Autodesk Fusion 360 part; units mm, degrees
note: some values were not read from the file. Chosen so that the rebuilt part matches the saved one: a side; which face or edge a step refers to. Set by a fixed rule: which sketch regions a step uses.
(part 2 of 2)
sketch "Sketch19" plane through (0, -4, 0) normal (0, -1, 0) x (1, 0, 0)
  line L0 (6.8, -6.4133) -> (7.8, -7.4133)
  line L1 (7.8, -7.4133) -> (11.75, -7.4133)
  line L2 (11.75, -7.4133) -> (11.75, -18.4133)
  line L3 (11.75, -18.4133) -> (0.75, -18.4133)
  line L4 (0.75, -18.4133) -> (0.75, -7.4133)
  line L5 (0.75, -7.4133) -> (4.7, -7.4133)
  line L6 (4.7, -7.4133) -> (5.7, -6.4133)
  line L7 (5.7, -6.4133) -> (5.7, 19.65)
  line L8 (5.7, 19.65) -> (6.8, 19.65)
  line L9 (6.8, 19.65) -> (6.8, -6.4133)
  arc A0 (25.83, 39.15) -> (20.83, 44.15) centre (20.83, 39.15) ccw
  line L10 (20.83, 44.15) -> (-20.83, 44.15)
  arc A1 (-20.83, 44.15) -> (-25.83, 39.15) centre (-20.83, 39.15) ccw
  line L11 (-25.83, 39.15) -> (-25.83, -22)
  arc A2 (-25.83, -22) -> (-20.83, -27) centre (-20.83, -22) ccw
  line L12 (-20.83, -27) -> (20.83, -27)
  arc A3 (20.83, -27) -> (25.83, -22) centre (20.83, -22) ccw
  line L13 (25.83, -22) -> (25.83, 39.15)
  line L14 (-15, 37.7778) -> (-15, 39)
  line L15 (-15, 39) -> (15, 39)
  line L16 (15, 39) -> (15, 37.7778)
  line L17 (15, 37.7778) -> (-15, 37.7778)
  circle A4 centre (20.83, 39.15) radius 1.5
  circle A5 centre (20.83, -22) radius 1.5
  circle A6 centre (-20.83, 39.15) radius 1.5
  circle A7 centre (-20.83, -22) radius 1.5
  line L18 (-5.7, -6.4133) -> (-4.7, -7.4133)
  line L19 (-4.7, -7.4133) -> (-0.75, -7.4133)
  line L20 (-0.75, -7.4133) -> (-0.75, -18.4133)
  line L21 (-0.75, -18.4133) -> (-11.75, -18.4133)
  line L22 (-11.75, -18.4133) -> (-11.75, -7.4133)
  line L23 (-11.75, -7.4133) -> (-7.8, -7.4133)
  line L24 (-7.8, -7.4133) -> (-6.8, -6.4133)
  line L25 (-6.8, -6.4133) -> (-6.8, 19.65)
  line L26 (-6.8, 19.65) -> (-5.7, 19.65)
  line L27 (-5.7, 19.65) -> (-5.7, -6.4133)
  line L28 (-6.8, -6.4133) -> (-5.7, -6.4133)
  line L29 (-8.8, -6.4133) -> (-8.8, 21.65) construction
  line L30 (-8.8, 21.65) -> (-3.7, 21.65) construction
  line L31 (-3.7, 21.65) -> (-3.7, -6.4133) construction
  line L32 (-8.8, -6.4133) -> (-8.8, -7.4133)
  line L33 (-3.7, -6.4133) -> (-3.7, -7.4133)
  line L34 (-7.8, -7.4133) -> (-4.7, -7.4133) construction
  line L35 (0, -27) -> (0, 44.15) construction
  line L36 (-3.7, -7.4133) -> (-8.8, -7.4133)
  line L37 (-8.8, -7.4133) -> (-8.8, 21.65)
  line L38 (-8.8, 21.65) -> (-3.7, 21.65)
  line L39 (-3.7, 21.65) -> (-3.7, -7.4133)
  line L40 (8.8, -7.4133) -> (8.8, 21.65)
  line L41 (8.8, 21.65) -> (3.7, 21.65)
  line L42 (3.7, 21.65) -> (3.7, -7.4133)
  line L43 (3.7, -7.4133) -> (8.8, -7.4133)
  line L44 (6.8, -6.4133) -> (5.7, -6.4133)
  dimension "d112" = -2
  constraint coincident L24.end L25.start
  constraint coincident L18.start L27.end
  constraint coincident L23 L32.end
  constraint perpendicular L23 L32
  constraint coincident L19 L33.end
  constraint perpendicular L19 L33
  constraint coincident L23.end L24.start
  constraint coincident L18.end L19.start
  constraint midpoint L12 L35.start
  constraint midpoint L10 L35.end
  constraint horizontal L36
  constraint vertical L37
  constraint horizontal L38
  constraint vertical L39
  constraint symmetric L24.end L35 L0.start
  constraint symmetric L18.start L35 L6.end
  constraint symmetric L29.end L35 L40.end
  constraint symmetric L33.end L35 L42.end
  constraint symmetric L35 L32.end L40.start
  constraint symmetric L35 L30.end L41.end
extrude "Extrude27" cut sketch "Sketch19" against normal blind 3.7 contours L0 L1 L5 L6 L7 L8 L9 L40 L41 L42 L43 | L0 L6 L43 L44 | L18 L19 L23 L24 L25 L26 L27 L32 L33 L36 L37 L38 L39 | L18 L24 L28 L36 bodies 1
sketch "Sketch20" plane through (0, -4, 0) normal (0, -1, 0) x (1, 0, 0)
  line L0 (-10.35, -9.8133) -> (-2.15, -9.8133)
  line L1 (-2.15, -9.8133) -> (-2.15, -15.7882)
  line L2 (-2.15, -15.7882) -> (-4.5853, -17.1099)
  line L3 (-4.5853, -17.1099) -> (-7.8571, -17.1099)
  line L4 (-7.8571, -17.1099) -> (-10.35, -15.7085)
  line L5 (-10.35, -15.7085) -> (-10.35, -9.8133)
  line L6 (-6.4, -6.579) -> (-7.6343, -7.8133)
  line L7 (-7.6343, -7.8133) -> (-11.35, -7.8133)
  line L8 (-11.35, -7.8133) -> (-11.35, -18.0133)
  line L9 (-11.35, -18.0133) -> (-1.15, -18.0133)
  line L10 (-1.15, -18.0133) -> (-1.15, -7.8133)
  line L11 (-1.15, -7.8133) -> (-4.8657, -7.8133)
  line L12 (-4.8657, -7.8133) -> (-6.1, -6.579)
  line L13 (-6.1, -6.579) -> (-6.4, -6.579)
  line L14 (3.7, -7.4133) -> (3.7, 21.65) construction
  line L15 (3.7, 21.65) -> (8.8, 21.65) construction
  line L16 (8.8, 21.65) -> (8.8, -7.4133) construction
  line L17 (8.8, -7.4133) -> (11.75, -7.4133) construction
  line L18 (11.75, -7.4133) -> (11.75, -18.4133) construction
  line L19 (11.75, -18.4133) -> (0.75, -18.4133) construction
  line L20 (0.75, -18.4133) -> (0.75, -7.4133) construction
  line L21 (0.75, -7.4133) -> (3.7, -7.4133) construction
  arc A0 (25.83, 39.15) -> (20.83, 44.15) centre (20.83, 39.15) ccw construction
  line L22 (20.83, 44.15) -> (-20.83, 44.15) construction
  arc A1 (-20.83, 44.15) -> (-25.83, 39.15) centre (-20.83, 39.15) ccw construction
  line L23 (-25.83, 39.15) -> (-25.83, -22) construction
  arc A2 (-25.83, -22) -> (-20.83, -27) centre (-20.83, -22) ccw construction
  line L24 (-20.83, -27) -> (20.83, -27) construction
  arc A3 (20.83, -27) -> (25.83, -22) centre (20.83, -22) ccw construction
  line L25 (25.83, -22) -> (25.83, 39.15) construction
  line L26 (-15, 37.7778) -> (-15, 39) construction
  line L27 (-15, 39) -> (15, 39) construction
  line L28 (15, 39) -> (15, 37.7778) construction
  line L29 (15, 37.7778) -> (-15, 37.7778) construction
  circle A4 centre (20.83, 39.15) radius 1.5 construction
  circle A5 centre (20.83, -22) radius 1.5 construction
  circle A6 centre (-20.83, 39.15) radius 1.5 construction
  circle A7 centre (-20.83, -22) radius 1.5 construction
  line L30 (-8.8, -7.4133) -> (-8.8, 21.65) construction
  line L31 (-8.8, 21.65) -> (-3.7, 21.65) construction
  line L32 (-3.7, 21.65) -> (-3.7, -7.4133) construction
  line L33 (-3.7, -7.4133) -> (-0.75, -7.4133) construction
  line L34 (-0.75, -7.4133) -> (-0.75, -18.4133) construction
  line L35 (-0.75, -18.4133) -> (-11.75, -18.4133) construction
  line L36 (-11.75, -18.4133) -> (-11.75, -7.4133) construction
  line L37 (-11.75, -7.4133) -> (-8.8, -7.4133) construction
  line L38 (-8.5, -7.4133) -> (-8.5, 21.35)
  line L39 (-8.5, 21.35) -> (-4, 21.35)
  line L40 (-4, 21.35) -> (-4, -7.4133)
  line L41 (-8.5, -7.4133) -> (-8.5, -7.8133) construction
  line L42 (-4, -7.4133) -> (-4, -7.8133) construction
  line L43 (-8.5, -7.4133) -> (-8.5, -7.8133)
  line L44 (-4, -7.4133) -> (-4, -7.8133)
  line L45 (-1.15, -7.8133) -> (-4, -7.8133)
  line L46 (-8.5, -7.8133) -> (-11.35, -7.8133)
  line L47 (0, -27) -> (0, 44.15) construction
  line L48 (4.8657, -7.8133) -> (6.1, -6.579)
  line L49 (6.1, -6.579) -> (6.4, -6.579)
  line L50 (6.4, -6.579) -> (7.6343, -7.8133)
  line L51 (7.6343, -7.8133) -> (11.35, -7.8133)
  line L52 (1.15, -7.8133) -> (4.8657, -7.8133)
  line L53 (4, -7.4133) -> (4, -7.8133)
  line L54 (4, 21.35) -> (4, -7.4133)
  line L55 (8.5, 21.35) -> (4, 21.35)
  line L56 (8.5, -7.4133) -> (8.5, 21.35)
  line L57 (8.5, -7.4133) -> (8.5, -7.8133)
  line L58 (8.5, -7.8133) -> (11.35, -7.8133)
  line L59 (1.15, -7.8133) -> (4, -7.8133)
  dimension "d115" = 0.3
  constraint coincident L7 L41.end
  constraint perpendicular L7 L41
  constraint coincident L11 L42.end
  constraint perpendicular L11 L42
  constraint coincident L10.end L11.start
  constraint coincident L7.end L8.start
  constraint midpoint L24 L47.start
  constraint midpoint L22 L47.end
  constraint symmetric L6.start L47 L49.end
  constraint symmetric L6.end L47 L50.end
  constraint symmetric L7.end L47 L51.end
  constraint symmetric L10.end L47 L52.start
  constraint symmetric L11.end L47 L48.start
  constraint symmetric L12.end L47 L48.end
  constraint symmetric L38.start L47 L56.start
  constraint symmetric L38.end L47 L55.start
  constraint symmetric L39.end L47 L54.start
  constraint symmetric L40.end L47 L53.start
  constraint symmetric L41.end L47 L57.end
  constraint symmetric L42.end L47 L53.end
extrude "Extrude28" add sketch "Sketch20" against normal blind 1.8 contours L6 L7 L11 L12 L13 L38 L39 L40 L43 L44 | L48 L49 L50 L51 L52 L53 L54 L55 L56 L57 bodies 6 7
sketch "Sketch21" plane through (0, 7, 0) normal (0, -1, 0) x (1, 0, 0)
  line L0 (-7.8, -7.4133) -> (-11.75, -7.4133)
  line L1 (-11.75, -7.4133) -> (-11.75, -18.4133)
  line L2 (-11.75, -18.4133) -> (-0.75, -18.4133)
  line L3 (-0.75, -18.4133) -> (-0.75, -7.4133)
  line L4 (-0.75, -7.4133) -> (-4.7, -7.4133)
  line L5 (-4.7, -7.4133) -> (-5.7, -6.4133)
  line L6 (-5.7, -6.4133) -> (-5.7, 0)
  line L7 (-5.7, 0) -> (-5.75, 0)
  line L8 (-5.75, 0) -> (-6.75, 0)
  line L9 (-6.75, 0) -> (-6.8, 0)
  line L10 (-6.8, 0) -> (-6.8, -6.4133)
  line L11 (-6.8, -6.4133) -> (-7.8, -7.4133)
  line L12 (3.7, -7.4133) -> (3.7, 21.65)
  line L13 (3.7, 21.65) -> (8.8, 21.65)
  line L14 (8.8, 21.65) -> (8.8, -7.4133)
  line L15 (8.8, -7.4133) -> (11.75, -7.4133)
  line L16 (11.75, -7.4133) -> (11.75, -18.4133)
  line L17 (11.75, -18.4133) -> (0.75, -18.4133)
  line L18 (0.75, -18.4133) -> (0.75, -7.4133)
  line L19 (0.75, -7.4133) -> (3.7, -7.4133)
  arc A0 (25.83, 39.15) -> (20.83, 44.15) centre (20.83, 39.15) ccw
  line L20 (20.83, 44.15) -> (-20.83, 44.15)
  arc A1 (-20.83, 44.15) -> (-25.83, 39.15) centre (-20.83, 39.15) ccw
  line L21 (-25.83, 39.15) -> (-25.83, -22)
  arc A2 (-25.83, -22) -> (-20.83, -27) centre (-20.83, -22) ccw
  line L22 (-20.83, -27) -> (20.83, -27)
  arc A3 (20.83, -27) -> (25.83, -22) centre (20.83, -22) ccw
  line L23 (25.83, -22) -> (25.83, 39.15)
  line L24 (-15, 37.7778) -> (-15, 39)
  line L25 (-15, 39) -> (15, 39)
  line L26 (15, 39) -> (15, 37.7778)
  line L27 (15, 37.7778) -> (-15, 37.7778)
  circle A4 centre (20.83, 39.15) radius 1.5
  circle A5 centre (20.83, -22) radius 1.5
  circle A6 centre (-20.83, 39.15) radius 1.5
  circle A7 centre (-20.83, -22) radius 1.5
  line L28 (-8.8, -7.4133) -> (-8.8, 21.65)
  line L29 (-8.8, 21.65) -> (-3.7, 21.65)
  line L30 (-3.7, 21.65) -> (-3.7, -7.4133)
  line L31 (-3.7, -7.4133) -> (-0.75, -7.4133)
  line L32 (-0.75, -7.4133) -> (-0.75, -18.4133)
  line L33 (-0.75, -18.4133) -> (-11.75, -18.4133)
  line L34 (-11.75, -18.4133) -> (-11.75, -7.4133)
  line L35 (-11.75, -7.4133) -> (-8.8, -7.4133)
  line L36 (0, -27) -> (0, 44.15) construction
  line L37 (-7.8, -7.4133) -> (-6.8, -6.4133)
  line L38 (-6.8, -6.4133) -> (-6.8, 19.65)
  line L39 (-6.8, 19.65) -> (-5.7, 19.65)
  line L40 (-5.7, 19.65) -> (-5.7, -6.4133)
  line L41 (-5.7, -6.4133) -> (-4.7, -7.4133)
  line L42 (-4.7, -7.4133) -> (-3.7, -7.4133)
  line L43 (-3.7, -7.4133) -> (-3.7, 21.65)
  line L44 (-3.7, 21.65) -> (-8.8, 21.65)
  line L45 (-8.8, 21.65) -> (-8.8, -7.4133)
  line L46 (-8.8, -7.4133) -> (-7.8, -7.4133)
  line L47 (-6.25, 19.65) -> (-6.25, -10.35) construction
  line L48 (-6.25, -10.35) -> (-6.25, -10.95) construction
  line L49 (-11.75, -10.95) -> (-0.75, -10.95)
  line L50 (11.75, -10.95) -> (0.75, -10.95)
  dimension "d118" = 30
  dimension "d119" = 0.6
  constraint midpoint L22 L36.start
  constraint midpoint L20 L36.end
  constraint midpoint L39 L47.start
  constraint perpendicular L39 L47
  constraint parallel L47 L48
  constraint coincident L34 L49.start
  constraint coincident L32 L49.end
  constraint perpendicular L32 L49
  constraint symmetric L36 L49.start L50.start
  constraint symmetric L36 L49.end L50.end
  measures "d118" distance of L47.start L47.end
  measures "d119" distance of L47.end L48.end
extrude "Extrude29" add sketch "Sketch21" along normal blind 3 contours L1 L2 L3 L32 L33 L34 L49 | L16 L17 L18 L50 bodies 1
sketch "Sketch22" plane through (0, -4, 0) normal (0, -1, 0) x (1, 0, 0)
  line L0 (-10.35, -9.8133) -> (-2.15, -9.8133)
  line L1 (-2.15, -9.8133) -> (-2.15, -15.7882)
  line L2 (-2.15, -15.7882) -> (-4.5853, -17.1099)
  line L3 (-4.5853, -17.1099) -> (-7.8571, -17.1099)
  line L4 (-7.8571, -17.1099) -> (-10.35, -15.7085)
  line L5 (-10.35, -15.7085) -> (-10.35, -9.8133)
  line L6 (-8.5, -7.8133) -> (-11.35, -7.8133)
  line L7 (-11.35, -7.8133) -> (-11.35, -18.0133)
  line L8 (-11.35, -18.0133) -> (-1.15, -18.0133)
  line L9 (-1.15, -18.0133) -> (-1.15, -7.8133)
  line L10 (-1.15, -7.8133) -> (-4, -7.8133)
  line L11 (-4, -7.8133) -> (-4, 21.35)
  line L12 (-4, 21.35) -> (-8.5, 21.35)
  line L13 (-8.5, 21.35) -> (-8.5, -7.8133)
  line L14 (-11.35, -7.8133) -> (-1.15, -7.8133)
  line L15 (-1.15, -7.8133) -> (-1.15, -18.0133)
  line L16 (-1.15, -18.0133) -> (-11.35, -18.0133)
  line L17 (-11.35, -18.0133) -> (-11.35, -7.8133)
  line L18 (3.7, -7.4133) -> (3.7, 21.65) construction
  line L19 (3.7, 21.65) -> (8.8, 21.65) construction
  line L20 (8.8, 21.65) -> (8.8, -7.4133) construction
  line L21 (8.8, -7.4133) -> (11.75, -7.4133) construction
  line L22 (11.75, -7.4133) -> (11.75, -18.4133) construction
  line L23 (11.75, -18.4133) -> (0.75, -18.4133) construction
  line L24 (0.75, -18.4133) -> (0.75, -7.4133) construction
  line L25 (0.75, -7.4133) -> (3.7, -7.4133) construction
  arc A0 (25.83, 39.15) -> (20.83, 44.15) centre (20.83, 39.15) ccw construction
  line L26 (20.83, 44.15) -> (-20.83, 44.15) construction
  arc A1 (-20.83, 44.15) -> (-25.83, 39.15) centre (-20.83, 39.15) ccw construction
  line L27 (-25.83, 39.15) -> (-25.83, -22) construction
  arc A2 (-25.83, -22) -> (-20.83, -27) centre (-20.83, -22) ccw construction
  line L28 (-20.83, -27) -> (20.83, -27) construction
  arc A3 (20.83, -27) -> (25.83, -22) centre (20.83, -22) ccw construction
  line L29 (25.83, -22) -> (25.83, 39.15) construction
  line L30 (-15, 37.7778) -> (-15, 39) construction
  line L31 (-15, 39) -> (15, 39) construction
  line L32 (15, 39) -> (15, 37.7778) construction
  line L33 (15, 37.7778) -> (-15, 37.7778) construction
  circle A4 centre (20.83, 39.15) radius 1.5 construction
  circle A5 centre (20.83, -22) radius 1.5 construction
  circle A6 centre (-20.83, 39.15) radius 1.5 construction
  circle A7 centre (-20.83, -22) radius 1.5 construction
  line L34 (-8.8, -7.4133) -> (-8.8, 21.65) construction
  line L35 (-8.8, 21.65) -> (-3.7, 21.65) construction
  line L36 (-3.7, 21.65) -> (-3.7, -7.4133) construction
  line L37 (-3.7, -7.4133) -> (-0.75, -7.4133) construction
  line L38 (-0.75, -7.4133) -> (-0.75, -18.4133) construction
  line L39 (-0.75, -18.4133) -> (-11.75, -18.4133) construction
  line L40 (-11.75, -18.4133) -> (-11.75, -7.4133) construction
  line L41 (-11.75, -7.4133) -> (-8.8, -7.4133) construction
  line L42 (-8.5, -7.4133) -> (-4, -7.4133)
  line L43 (-8.5, -7.4133) -> (-8.5, -7.8133)
  line L44 (-4, -7.4133) -> (-4, -7.8133)
  line L45 (0, -27) -> (0, 44.15) construction
  line L46 (1.15, -18.0133) -> (11.35, -18.0133)
  line L47 (11.35, -18.0133) -> (11.35, -7.8133)
  line L48 (1.15, -7.8133) -> (1.15, -18.0133)
  line L49 (11.35, -7.8133) -> (1.15, -7.8133)
  line L50 (8.5, -7.4133) -> (8.5, -7.8133)
  line L51 (4, -7.4133) -> (4, -7.8133)
  line L52 (8.5, -7.4133) -> (4, -7.4133)
  constraint horizontal L14
  constraint vertical L15
  constraint horizontal L16
  constraint vertical L17
  constraint coincident L8.end L9.start
  constraint coincident L6.end L7.start
  constraint coincident L13 L42.start
  constraint coincident L11 L42.end
  constraint perpendicular L11 L42
  constraint coincident L6.start L13.end
  constraint perpendicular L6 L43
  constraint coincident L10.end L11.start
  constraint perpendicular L10 L44
  constraint midpoint L28 L45.start
  constraint midpoint L26 L45.end
  constraint symmetric L6.end L45 L47.end
  constraint symmetric L9.end L45 L48.start
  constraint symmetric L8.end L45 L46.start
  constraint symmetric L7.end L45 L46.end
  constraint symmetric L42.start L45 L50.start
  constraint symmetric L42.end L45 L51.start
  constraint symmetric L6.start L45 L50.end
  constraint symmetric L10.end L45 L51.end
extrude "Extrude30" cut sketch "Sketch22" against normal blind 3.5 contours L6 L7 L8 L9 L10 L14 L15 L16 L17 | L11 L13 L14 L42 L43 L44 | L46 L47 L48 L49 | L49 L50 L51 L52 bodies 6 7
move_body "Move2" bodies 6 to x (1, 0, 0) y (0, 1, 0) z (0, 0, 1) at (0, -20, 0)
sketch "Sketch23" plane through (0, 0, -7.4133) normal (0, 0, -1) x (-1, 0, 0)
  line L0 (5.2657, -20.5) -> (5.2657, -22.2)
  line L1 (5.2657, -22.2) -> (4, -22.2)
  line L2 (4, -22.2) -> (4, -24)
  line L3 (4, -24) -> (8.5, -24)
  line L4 (8.5, -24) -> (8.5, -22.2)
  line L5 (8.5, -22.2) -> (7.2343, -22.2)
  line L6 (7.2343, -22.2) -> (7.2343, -20.5)
  line L7 (7.2343, -20.5) -> (5.2657, -20.5)
  line L8 (7.2343, -22.2) -> (5.2657, -22.2)
  line L9 (5.2657, -22.2) -> (5.2657, -20.5)
  line L10 (5.2657, -20.5) -> (7.2343, -20.5)
  line L11 (7.2343, -20.5) -> (7.2343, -22.2)
  constraint horizontal L8
  constraint vertical L9
  constraint horizontal L10
  constraint vertical L11
  constraint coincident L0.start L7.end
  constraint coincident L5.end L6.start
extrude "Extrude31" cut sketch "Sketch23" against normal blind 5 contours L0 L6 L7 L8 L9 L10 L11 bodies 6
extrude "Extrude32" add 1 faces at (-7, -22.2, 11.7622) along direction (0, 1, 0) blind 1.88 on bodies 6 bodies 6
move_body "Move3" bodies 6 to x (1, 0, 0) y (0, 1, 0) z (0, 0, 1) at (0, 20, 0)
sketch "Sketch24" plane through (0, -4, 0) normal (0, -1, 0) x (1, 0, 0)
  line L0 (-8.5, -7.4133) -> (-4, -7.4133)
  line L1 (-4, -7.4133) -> (-4, 21.35)
  line L2 (-4, 21.35) -> (-8.5, 21.35)
  line L3 (-8.5, 21.35) -> (-8.5, -7.4133)
  line L4 (-7.8, -7.4133) -> (-6.8, -6.4133)
  line L5 (-6.8, -6.4133) -> (-6.8, 19.65)
  line L6 (-6.8, 19.65) -> (-5.7, 19.65)
  line L7 (-5.7, 19.65) -> (-5.7, -6.4133)
  line L8 (-5.7, -6.4133) -> (-4.7, -7.4133)
  line L9 (-4.7, -7.4133) -> (-3.7, -7.4133)
  line L10 (-3.7, -7.4133) -> (-3.7, 21.65)
  line L11 (-3.7, 21.65) -> (-8.8, 21.65)
  line L12 (-8.8, 21.65) -> (-8.8, -7.4133)
  line L13 (-8.8, -7.4133) -> (-7.8, -7.4133)
  line L14 (-6.8, -6.4133) -> (-5.7, -6.4133)
  constraint coincident L4.end L5.start
  constraint coincident L7.end L8.start
extrude "Extrude33" cut sketch "Sketch24" against normal blind 3.68 contours L0 L4 L8 L14 bodies 6
hidden bodies 2 3 4 5 7
equation "d113 = -2 mm + ( -1.7 mm )"
named bodies: "body", "terminal", "terminal (1)", "cover", "Terminal Certo", "Cable Holder 1", "Cable Holder 2"
